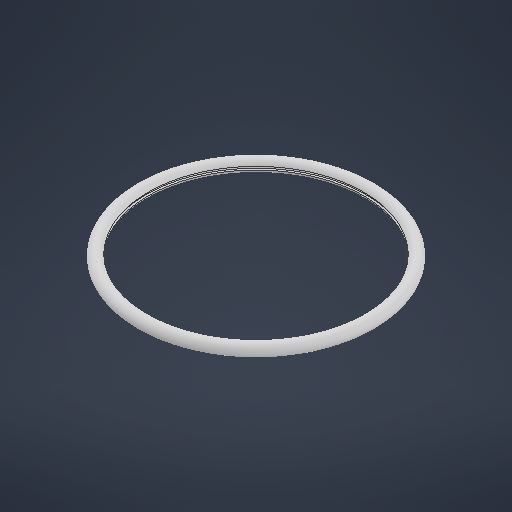
# Autodesk Inventor part: foam_bumper_circular
Saved by Autodesk Inventor 2026 (Build 300175050, 175E)
## iProperties
Created: 2025-06-14
Part Number: foam_bumper_circular
Material: Generic
Document SubType Name: Modeling
Designer: satom
Density: 1 g/cm^3
Appearance: Default
Author: satom
Autodesk Inventor part; units mm, degrees
ref_plane "YZ Plane" through (0, 0, 0) normal (1, 0, 0) x (0, 1, 0)
ref_plane "XZ Plane" through (0, 0, 0) normal (0, 1, 0) x (-1, 0, 0)
ref_plane "XY Plane" through (0, 0, 0) normal (0, 0, 1) x (1, 0, 0)
sketch "Sketch1" plane through (0, 0, 0) normal (1, 0, 0) x (0, 1, 0)
  line L0 (0, 181.8065) -> (0, 79.5332) construction
  line L1 (0, 90.7423) -> (0, 123.3903) construction
  arc A0 (2.5, 167.8089) -> (-2.5, 167.8089) centre (0, 177) ccw
  arc A1 (2.5, 171.1628) -> (-2.5, 171.1628) centre (0, 177) ccw
  line L2 (2.5, 171.1628) -> (2.5, 167.8089)
  line L3 (-2.5, 171.1628) -> (-2.5, 167.8089)
  line L4 (0, 0) -> (39.543, 0) construction
  dimension "d5" = 19.05
  dimension "d6" = 12.7
  dimension "d7" = 5
  dimension "d8" = 2.5
  dimension "d9" = 177
  constraints: 10 end point, 5 vertical, 4 point on circle, 2 centre point, 2 horizontal, 1 coincident, 1 collinear, 1 point on line
  measures "d5" diameter of A0
  measures "d6" diameter of A1
  measures "d7" distance between parallel lines of L3 L2
  measures "d8" distance between parallel lines of L0 L2
  measures "d9" distance from line of L4 A0.centre
revolve "Revolution1" add sketch "Sketch1" angle 360 about axis through (0, 0, 0) along (0, 1, 0)
equation "\"d7\" = hardboard_thickness"
equation "\"d8\" = 0.5 * hardboard_thickness"
equation "\"d9\" = 0.5 * robot_diameter"
equation "\"m3_heat_set_insert\" = 4"
equation "\"m3_clearance\" = 3.4"
equation "\"m3_heat_set_depth\" = 7"
equation "\"robot_diameter\" = 354"
equation "\"hardboard_thickness\" = 5"
equation "\"motor_centerline_height\" = 13"
body "Solid1"
